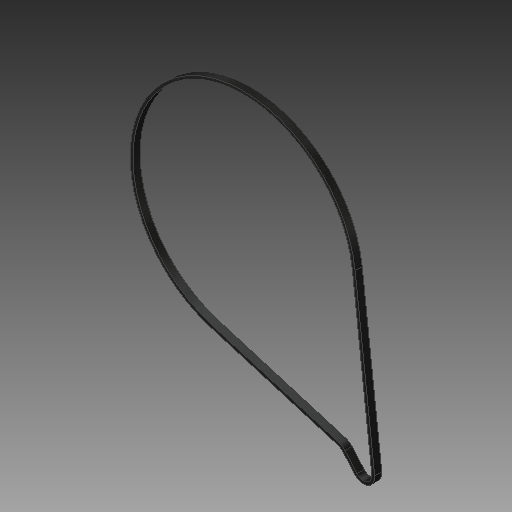
# Autodesk Inventor part: CarouselBelt
Saved by Autodesk Inventor 2018 (Build 220112000, 112)
## iProperties
Created: 2020-02-05
Part Number: CarouselBelt
Material: Generic
Document SubType Name: Modeling
Designer: Myers
Mass: 80.2665 g
Surface Area: 470.855 cm^2
Volume: 80.2665 cm^3
Density: 1 g/cm^3
Appearance: Black Cast
Author: Myers
Autodesk Inventor part; units mm, degrees
ref_plane "YZ Plane" through (0, 0, 0) normal (1, 0, 0) x (0, 1, 0)
ref_plane "XZ Plane" through (0, 0, 0) normal (0, 1, 0) x (-1, 0, 0)
ref_plane "XY Plane" through (0, 0, 0) normal (0, 0, 1) x (1, 0, 0)
sketch "Sketch1" plane through (0, 0, 0) normal (0, 0, 1) x (1, 0, 0)
  circle A0 centre (0, 0) radius 19.1008 construction
  circle A1 centre (-47.625, 0) radius 16.9418 construction
  circle A2 centre (-203.2, 263.525) radius 190.5 construction
  arc A3 (-13.9752, 285.5302) -> (-258.155, 81.1238) centre (-203.2, 263.525) ccw
  line L0 (-13.9752, 285.5302) -> (18.9729, 2.2064)
  line L1 (-42.7377, 16.2215) -> (-258.155, 81.1238)
  arc A4 (-34.8034, 11.0739) -> (-42.7377, 16.2215) centre (-47.625, 0) ccw
  arc A5 (-14.4555, -12.4852) -> (18.9729, 2.2064) centre (0, 0) ccw
  line L2 (-34.8034, 11.0739) -> (-14.4555, -12.4852)
  arc A6 (-10.8512, -9.3722) -> (14.2423, 1.6563) centre (0, 0) ccw
  line L3 (-10.8512, -9.3722) -> (-31.1992, 14.1869)
  arc A7 (-31.1992, 14.1869) -> (-41.3638, 20.7816) centre (-47.625, 0) ccw
  line L4 (-41.3638, 20.7816) -> (-256.7811, 85.6838)
  arc A8 (-18.7058, 284.9801) -> (-256.7811, 85.6838) centre (-203.2, 263.525) ccw
  line L5 (-18.7058, 284.9801) -> (14.2423, 1.6563)
  dimension "d0" = 381
  dimension "d1" = 33.8836
  dimension "d2" = 38.2016
  dimension "d3" = 155.575
  dimension "d4" = 203.2
  dimension "d5" = 263.525
  dimension "d6" = 4.7625
  constraints: 12 end point, 12 point on circle, 9 centre point, 6 concentric, 6 tangent, 1 coincident, 1 horizontal alignment, 5 other
  measures "d0" diameter of A2
  measures "d1" diameter of A1
  measures "d2" diameter of A0
  measures "d3" horizontal distance of A1.centre A2.centre
  measures "d4" horizontal distance of point (0, 0) A2.centre
  measures "d5" vertical distance of A2.centre point (0, 0)
  measures "d6" radial gap between concentric circles of A2 A8
extrude "Extrusion1" add sketch "Sketch1" along normal mid plane 12
body "Solid1"
